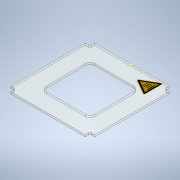
# Autodesk Inventor part: Schutzglas_oben
Saved by Autodesk Inventor 2022 (Build 260153000, 153)
## iProperties
Created: 2021-04-25
Part Number: Schutzglas_oben
Material: Glas
Document SubType Name: Modeling
Designer: Sebastian Seewald
Mass: 394.504 g
Surface Area: 938.858 cm^2
Volume: 180.965 cm^3
Density: 2.18 g/cm^3
Appearance: Klar
Author: Sebastian Seewald
Autodesk Inventor part; units mm, degrees
ref_plane "YZ Plane" through (0, 0, 0) normal (1, 0, 0) x (0, 1, 0)
ref_plane "XZ Plane" through (0, 0, 0) normal (0, 1, 0) x (-1, 0, 0)
ref_plane "XY Plane" through (0, 0, 0) normal (0, 0, 1) x (1, 0, 0)
sketch "Skizze1" plane through (0, 0, 0) normal (0, 0, 1) x (1, 0, 0)
  line L0 (-86.35, 2) -> (86.35, 2)
  line L1 (86.35, 2) -> (86.35, -2)
  line L2 (86.35, -2) -> (-86.35, -2)
  line L3 (-86.35, -2) -> (-86.35, 2)
  line L4 (-86.35, 2) -> (86.35, -2) construction
  line L5 (86.35, 2) -> (-86.35, -2) construction
  point P0 (0, 0)
  dimension "d0" = 4
  dimension "d1" = 172.7
  constraints: 12 end point, 2 midpoint, 2 parallel, 1 horizontal, 1 perpendicular
  measures "d0" distance of L2.end L0.start
  measures "d1" distance between parallel lines of L3 L1
extrude "Extrusion1" add sketch "Skizze1" along normal blind 172.7
sketch "Skizze2" plane through (-86.35, -2, 0) normal (0, -1, 0) x (1, 0, 0)
  line L0 (172.7, 0) -> (172.7, 172.7) projected
  line L1 (46.35, 136.35) -> (126.35, 136.35)
  line L2 (136.35, 126.35) -> (136.35, 46.35)
  line L3 (126.35, 36.35) -> (46.35, 36.35)
  line L4 (36.35, 46.35) -> (36.35, 126.35)
  line L5 (172.7, 0) -> (0, 0) projected
  line L6 (0, 0) -> (0, 172.7) projected
  line L7 (172.7, 172.7) -> (0, 172.7) projected
  arc A0 (46.35, 136.35) -> (36.35, 126.35) centre (46.35, 126.35) ccw
  arc A1 (36.35, 46.35) -> (46.35, 36.35) centre (46.35, 46.35) ccw
  arc A2 (126.35, 36.35) -> (136.35, 46.35) centre (126.35, 46.35) ccw
  arc A3 (136.35, 126.35) -> (126.35, 136.35) centre (126.35, 126.35) ccw
  point P0 (86.35, 0)
  point P1 (36.35, 136.35)
  point P2 (136.35, 136.35)
  point P3 (36.35, 36.35)
  dimension "d50" = 100
  dimension "d51" = 100
  dimension "d52" = 36.35
  dimension "d53" = 36.35
  dimension "d54" = 36.35
  dimension "d55" = 36.35
  dimension "d56" = 10
  constraints: 8 end point, 8 point on circle, 8 tangent, 6 point on line, 4 centre point, 3 equal radius, 2 parallel, 1 horizontal, 1 perpendicular
  measures "d50" distance of point (36.35, 36.35) point (36.35, 136.35)
  measures "d51" distance of point (36.35, 136.35) point (136.35, 136.35)
  measures "d52" distance between parallel lines of L5 L3
  measures "d53" distance between parallel lines of L0 L2
  measures "d54" distance between parallel lines of L6 L4
  measures "d55" distance between parallel lines of L7 L1
  measures "d56" radius of A0
extrude "Extrusion2" cut sketch "Skizze2" against normal blind 10 contours L1 A3 L2 A2 L3 A1 L4 A0
sketch "Skizze3" plane through (-86.35, 2, 0) normal (0, 1, 0) x (1, 0, 0)
  line L0 (114.5855, -0.5055) -> (156.5746, -0.5055) construction
  line L1 (156.5746, -0.5055) -> (156.5746, -42.4946) construction
  line L2 (156.5746, -42.4946) -> (114.5855, -42.4946) construction
  line L3 (114.5855, -42.4946) -> (114.5855, -0.5055) construction
  point P0 (86.35, 0)
  dimension "d1" = 172.7
  constraints: 2 other
sketch "Skizze4" plane through (-86.35, 2, 0) normal (0, 1, 0) x (1, 0, 0)
  line L0 (0, -172.7) -> (172.7, -172.7) projected
  line L1 (0, -172.7) -> (10, -172.7)
  line L2 (10, -172.7) -> (10, -162.7)
  line L3 (10, -162.7) -> (0, -162.7)
  line L4 (0, -162.7) -> (0, -172.7)
  line L5 (0, 0) -> (0, -172.7) projected
  line L6 (0, 0) -> (10, 0)
  line L7 (10, 0) -> (10, -10)
  line L8 (10, -10) -> (0, -10)
  line L9 (0, -10) -> (0, 0)
  line L10 (172.7, 0) -> (162.7, 0)
  line L11 (162.7, 0) -> (162.7, -10)
  line L12 (162.7, -10) -> (172.7, -10)
  line L13 (172.7, -10) -> (172.7, 0)
  line L14 (172.7, 0) -> (172.7, -172.7) projected
  line L15 (172.7, -172.7) -> (162.7, -172.7)
  line L16 (162.7, -172.7) -> (162.7, -162.7)
  line L17 (162.7, -162.7) -> (172.7, -162.7)
  line L18 (172.7, -162.7) -> (172.7, -172.7)
  line L19 (172.7, 0) -> (0, 0) projected
  point P0 (86.35, 0)
  point P1 (0, -10)
  dimension "d57" = 10
  dimension "d58" = 10
  dimension "d59" = 10
  dimension "d60" = 10
  dimension "d61" = 10
  dimension "d62" = 10
  dimension "d63" = 10
  constraints: 32 end point, 8 parallel, 4 horizontal, 4 perpendicular, 1 point on line
  measures "d57" distance between parallel lines of L0 L3
  measures "d58" distance between parallel lines of L5 L2
  measures "d59" distance between parallel lines of L19 L8
  measures "d60" distance between parallel lines of L5 L7
  measures "d61" distance between parallel lines of L0 L17
  measures "d62" distance between parallel lines of L14 L16
  measures "d63" distance between parallel lines of L14 L11
extrude "Extrusion3" cut sketch "Skizze4" against normal blind 10 contours L4 L3 L2 L0 | L16 L17 L14 L0 | L5 L6 L7 L8 | L12 L11 L10 L13
fillet "Rundung1" radius 4 4 edges at (76.35, 0, 162.7) (76.35, 0, 10) (-76.35, 0, 10) (-76.35, 0, 162.7)
